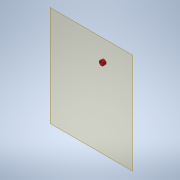
# Autodesk Inventor part: ball screw end thrust bearing
Saved by Autodesk Inventor 2020 (Build 240168000, 168)
## iProperties
Created: 2020-07-30
Part Number: ball screw end thrust bearing
Material: Generic
Document SubType Name: Modeling
Designer: Vikki
Mass: 2.35619 g
Surface Area: 14.1372 cm^2
Volume: 2.35619 cm^3
Density: 1 g/cm^3
Appearance: Light Red
Author: Vikki
Autodesk Inventor part; units mm, degrees
ref_plane "YZ Plane" through (0, 0, 0) normal (1, 0, 0) x (0, 1, 0)
ref_plane "XZ Plane" through (0, 0, 0) normal (0, 1, 0) x (-1, 0, 0)
ref_plane "XY Plane" through (0, 0, 0) normal (0, 0, 1) x (1, 0, 0)
ref_plane "Work Plane1" through (0, 0, 0) normal (0, 0, 1) x (1, 0, 0)
sketch "Sketch1" plane through (0, 0, 0) normal (0, 0, 1) x (1, 0, 0)
  circle A0 centre (161, 121) radius 10
  circle A1 centre (161, 121) radius 5
  point P0 (0, 0)
  dimension "d0" = 20
  dimension "d1" = 10
  constraints: 2 centre point, 1 coincident
  measures "d0" diameter of A0
  measures "d1" diameter of A1
extrude "Extrusion1" add sketch "Sketch1" along normal blind 10
body "Solid1"
